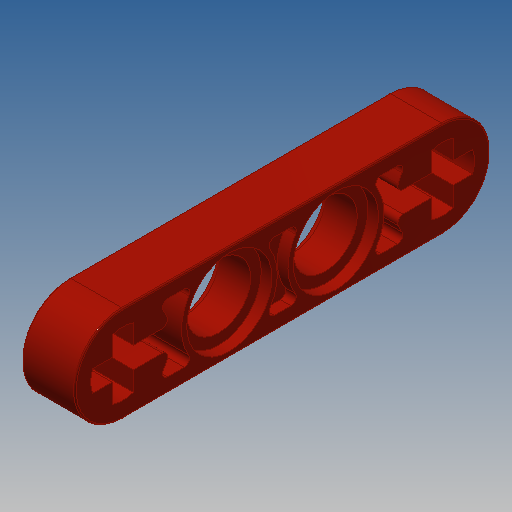
# Autodesk Inventor part: 32449-Red
Saved by Autodesk Inventor 2022.2 (Build 262287000, 287)
## iProperties
Created: 2012-03-28
Part Number: 32449-Red
Document SubType Name: Modeling
Designer: D. Kohfeld
Density: 1.06 g/cm^3
Material: ABS Plastic
Mass: 0.517 g
Surface Area: 9.49423 cm^2
Volume: 0.487736 cm^3
Appearance: Red
Author: D. Kohfeld
Autodesk Inventor part; units mm, degrees
ref_plane "YZ Plane" through (0, 0, 0) normal (1, 0, 0) x (0, 1, 0)
ref_plane "XZ Plane" through (0, 0, 0) normal (0, 1, 0) x (-1, 0, 0)
ref_plane "XY Plane" through (0, 0, 0) normal (0, 0, 1) x (1, 0, 0)
sketch "Sketch3" plane through (0, 0, 0) normal (1, 0, 0) x (0, 1, 0)
  arc A0 (12.8, 2.2627) -> (11.2, 2.2627) centre (12, 0) ccw
  arc A1 (11.2, -2.2627) -> (12.8, -2.2627) centre (12, 0) ccw
  arc A2 (14.2627, -0.8) -> (14.2627, 0.8) centre (12, 0) ccw
  line L0 (14.2627, 0.8) -> (12.8, 0.8)
  line L1 (11.2, 0.8) -> (8.49, 0.8)
  line L2 (12.8, 2.2627) -> (12.8, 0.8)
  line L3 (12.8, -0.8) -> (12.8, -2.2627)
  line L4 (14.2627, -0.8) -> (12.8, -0.8)
  line L5 (11.2, -0.8) -> (8.49, -0.8)
  arc A3 (12, -3.6) -> (12, 3.6) centre (12, 0) ccw
  line L6 (-12, -3.6) -> (12, -3.6)
  line L7 (-12, 3.6) -> (12, 3.6)
  line L8 (11.2, 0.8) -> (11.2, 2.2627)
  line L9 (11.2, -0.8) -> (11.2, -2.2627)
  arc A4 (-12, 3.6) -> (-12, -3.6) centre (-12, 0) ccw
  line L10 (0, -3.6) -> (0, 3.6) construction
  arc A5 (-11.2, 2.2627) -> (-12.8, 2.2627) centre (-12, 0) ccw
  arc A6 (-12.8, -2.2627) -> (-11.2, -2.2627) centre (-12, 0) ccw
  line L11 (-12.8, -0.8) -> (-12.8, -2.2627)
  line L12 (-12.8, 2.2627) -> (-12.8, 0.8)
  line L13 (-14.2627, -0.8) -> (-12.8, -0.8)
  line L14 (-14.2627, 0.8) -> (-12.8, 0.8)
  arc A7 (-14.2627, 0.8) -> (-14.2627, -0.8) centre (-12, 0) ccw
  line L15 (-11.2, 0.8) -> (-8.49, 0.8)
  line L16 (-11.2, -0.8) -> (-8.49, -0.8)
  line L17 (-11.2, 0.8) -> (-11.2, 2.2627)
  line L18 (-11.2, -0.8) -> (-11.2, -2.2627)
  circle A8 centre (-4, 0) radius 3.2
  circle A9 centre (4, 0) radius 3.2
  line L19 (12, 0) -> (4, 0) construction
  line L20 (4, 0) -> (-4, 0) construction
  line L21 (-4, 0) -> (-12, 0) construction
  circle A10 centre (-4, 0) radius 2.4
  circle A11 centre (4, 0) radius 2.4
  line L22 (-9.4544, 2.5456) -> (-6.5456, 2.5456)
  line L23 (-9.4544, -2.5456) -> (-6.5456, -2.5456)
  line L24 (-1.4544, 2.5456) -> (1.4544, 2.5456)
  line L25 (-1.4544, -2.5456) -> (1.4544, -2.5456)
  line L26 (6.5456, 2.5456) -> (9.4544, 2.5456)
  line L27 (6.5456, -2.5456) -> (9.4544, -2.5456)
  arc A12 (-9.4544, -2.5456) -> (-9.4544, 2.5456) centre (-12, 0) ccw
  arc A13 (-6.5456, 2.5456) -> (-6.5456, -2.5456) centre (-4, 0) ccw
  arc A14 (-1.4544, -2.5456) -> (-1.4544, 2.5456) centre (-4, 0) ccw
  arc A15 (1.4544, 2.5456) -> (1.4544, -2.5456) centre (4, 0) ccw
  arc A16 (6.5456, -2.5456) -> (6.5456, 2.5456) centre (4, 0) ccw
  arc A17 (9.4544, 2.5456) -> (9.4544, -2.5456) centre (12, 0) ccw
  line L28 (-12, 0) -> (-9.4544, 2.5456) construction
  arc A18 (8.49, 0.8) -> (8.49, -0.8) centre (12, 0) ccw
  point P0 (0, 0)
  dimension "d47" = 4.8
  dimension "d49" = 7.2
  dimension "d53" = 1.6
  dimension "d58" = 24
  dimension "d59" = 6.4
  dimension "d60" = 4.8
  dimension "d64" = 45
  constraints: 58 end point, 32 point on circle, 19 centre point, 14 symmetric about line, 11 equal radius, 11 parallel, 10 coincident, 8 equal length, 7 horizontal alignment, 6 perpendicular, 4 tangent, 2 collinear, 2 horizontal, 2 midpoint, 1 vertical, 1 vertical alignment, 3 other
  measures "d47" diameter of A1
  measures "d49" diameter of A3
  measures "d53" distance between parallel lines of L0 L4
  measures "d58" distance of A0.centre A4.centre
  measures "d59" diameter of A8
  measures "d60" diameter of A10
  measures "d64" angle of L15 L28
extrude "Extrusion4" add sketch "Sketch3" along normal mid plane 4 contours L6 A4 L7 A3 | A8 | A9 | L24 A15 L25 A14
sketch "Sketch11" plane through (2, 0, 0) normal (1, 0, 0) x (0, 0, -1)
  circle A0 centre (0, 4) radius 2.4 projected
  circle A1 centre (0, -4) radius 2.4 projected
  circle A2 centre (0, 4) radius 3.2
  circle A3 centre (0, -4) radius 3.2
  arc A4 (2.5456, 6.5456) -> (-2.5456, 6.5456) centre (0, 4) ccw projected
  arc A5 (-2.5456, -6.5456) -> (2.5456, -6.5456) centre (0, -4) ccw projected
  line L0 (-2.2627, -11.2) -> (-0.8, -11.2) projected
  line L1 (-2.5456, 1.4544) -> (-2.5456, -1.4544)
  line L2 (2.5456, 1.4544) -> (2.5456, -1.4544)
  arc A6 (-2.5456, 1.4544) -> (2.5456, 1.4544) centre (0, 4) ccw
  arc A7 (2.5456, -1.4544) -> (-2.5456, -1.4544) centre (0, -4) ccw
  point P0 (0, 0)
  dimension "d61" = 6.4
  constraints: 4 centre point, 4 coincident, 4 end point, 4 point on circle, 3 equal radius, 2 vertical alignment, 1 parallel, 1 perpendicular
  measures "d61" diameter of A3
extrude "Extrusion16" cut sketch "Sketch11" against normal blind 0.8 contours A2 | A3
extrude "Extrusion17" cut sketch "Sketch11" against normal blind 0.8 contours A6 L2 A7 L1
mirror "Mirror3" about plane through (0, 0, 0) normal (1, 0, 0) of "Extrusion16", "Extrusion17"
fillet "Fillet1" radius 0.1 8 edges at (-2, 15.6, 0) (-2, 0, 3.6) (-2, 0, -3.6) (2, 0, 3.6) (2, 0, -3.6) (2, 15.6, 0) (2, -15.6, 0) (-2, -15.6, 0)
fillet "Fillet1" radius 0.4 20 edges at (0, -9.4544, 2.5456) (0, -6.5456, 2.5456) (0, -9.4544, -2.5456) (0, -6.5456, -2.5456) (0, 6.5456, 2.5456) (0, 9.4544, 2.5456) (0, 6.5456, -2.5456) (0, 9.4544, -2.5456) (1.6, -1.4544, 2.5456) (1.6, 1.4544, 2.5456) (1.6, -1.4544, -2.5456) (1.6, 1.4544, -2.5456) (-1.6, -1.4544, 2.5456) (-1.6, 1.4544, 2.5456) (-1.6, -1.4544, -2.5456) (-1.6, 1.4544, -2.5456) (0, -8.49, 0.8) (0, -8.49, -0.8) (0, 8.49, -0.8) (0, 8.49, 0.8)
equation "\"d47\" = kd"
equation "\"d49\" = tlad"
equation "\"d53\" = axlet"
equation "\"d58\" = 3 * lu"
equation "\"d59\" = tsd"
equation "\"d60\" = tpd"
equation "\"d15\" = 0.5 * lu"
equation "\"d61\" = tsd"
equation "\"d62\" = tsl"
equation "\"d65\" = 0.5 * lu - 2 * wall"
equation "\"d56\" = lf"
equation "\"d67\" = tf"
equation "\"lf\" = 0.1"
equation "\"tf\" = 0.4"
equation "\"kd\" = 4.8"
equation "\"tlad\" = 7.2"
equation "\"axlet\" = 1.6"
equation "\"lu\" = 8"
equation "\"tsd\" = 6.4"
equation "\"tpd\" = 4.8"
equation "\"tsl\" = 0.8"
equation "\"wall\" = 1.6"
body "Solid1"
